Autodesk Fusion 360 part; units mm, degrees
(part 2 of 3)
sketch "스케치1 (3)" plane through (0, 0, 0) normal (0, 0, 1) x (1, 0, 0) in component "rightKey2"
  line L0 (104.5156, 0) -> (228.5, 0)
  line L1 (150.5375, 25.575) -> (136.5375, 25.575)
  line L2 (160.0625, 44.625) -> (146.0625, 44.625)
  line L3 (145.775, 6.525) -> (131.775, 6.525)
  line L4 (145.775, 20.525) -> (145.775, 6.525)
  line L5 (150.825, 6.525) -> (150.825, 20.525)
  line L6 (131.775, 20.525) -> (145.775, 20.525)
  line L7 (126.725, 20.525) -> (126.725, 6.525)
  line L8 (150.5375, 39.575) -> (150.5375, 25.575)
  line L9 (131.4875, 39.575) -> (131.4875, 25.575)
  line L10 (136.5375, 39.575) -> (150.5375, 39.575)
  line L11 (177.0187, 44.625) -> (177.0187, 50.525)
  line L12 (175.5187, 57.225) -> (175.5187, 52.725)
  line L13 (126.725, 82.725) -> (112.725, 82.725)
  line L14 (112.725, 96.725) -> (126.725, 96.725)
  line L15 (164.825, 20.525) -> (164.825, 6.525)
  line L16 (127.0125, 44.625) -> (127.0125, 58.625)
  line L17 (221.975, 58.625) -> (221.975, 44.625)
  line L18 (124.4875, 42.1) -> (124.4875, 61.15)
  line L19 (119.725, 61.15) -> (124.4875, 61.15)
  line L20 (126.725, 6.525) -> (112.725, 6.525)
  line L21 (191.0188, 58.625) -> (191.0188, 52.725)
  line L22 (146.0625, 44.625) -> (146.0625, 58.625)
  line L23 (192.5187, 52.725) -> (192.5187, 57.225)
  line L24 (129.25, 0) -> (129.25, 103.25) construction
  line L25 (177.0187, 52.725) -> (177.0188, 58.625)
  line L26 (207.975, 44.625) -> (207.975, 58.625)
  line L27 (169.875, 6.525) -> (169.875, 20.525)
  line L28 (188.925, 20.525) -> (202.925, 20.525)
  line L29 (175.5188, 46.025) -> (168.7188, 46.025)
  line L30 (162.7313, 25.575) -> (162.7313, 39.575)
  line L31 (141.0125, 58.625) -> (141.0125, 44.625)
  line L32 (160.0625, 58.625) -> (160.0625, 44.625)
  line L33 (207.975, 6.525) -> (207.975, 20.525)
  line L34 (191.0188, 44.625) -> (177.0187, 44.625)
  line L35 (228.5, 103.25) -> (110.2, 103.25)
  line L36 (221.975, 25.575) -> (207.975, 25.575)
  line L37 (176.7313, 39.575) -> (176.7313, 25.575)
  line L38 (202.925, 25.575) -> (188.925, 25.575)
  line L39 (202.925, 6.525) -> (188.925, 6.525)
  line L40 (141.0125, 44.625) -> (127.0125, 44.625)
  line L41 (136.5375, 25.575) -> (136.5375, 39.575)
  line L42 (131.775, 6.525) -> (131.775, 20.525)
  line L43 (112.725, 20.525) -> (126.725, 20.525)
  line L44 (175.5188, 50.525) -> (175.5188, 46.025)
  line L45 (221.975, 39.575) -> (221.975, 25.575)
  line L46 (114.9625, 42.1) -> (124.4875, 42.1)
  line L47 (177.0187, 50.525) -> (175.5188, 50.525)
  line L48 (117.4875, 39.575) -> (131.4875, 39.575)
  line L49 (131.4875, 25.575) -> (117.4875, 25.575)
  line L50 (188.925, 39.575) -> (202.925, 39.575)
  line L51 (162.7313, 39.575) -> (176.7313, 39.575)
  line L52 (177.0188, 58.625) -> (191.0188, 58.625)
  line L53 (177.9, 90.825) -> (179.4, 90.825)
  line L54 (136.25, 63.675) -> (122.25, 63.675)
  line L55 (155.3, 63.675) -> (141.3, 63.675)
  line L56 (207.975, 96.725) -> (221.975, 96.725)
  line L57 (145.775, 82.725) -> (131.775, 82.725)
  line L58 (179.4, 96.725) -> (193.4, 96.725)
  circle A0 centre (225.4, 3.1) radius 1.6
  line L59 (122.25, 63.675) -> (122.25, 77.675)
  line L60 (127.0125, 58.625) -> (141.0125, 58.625)
  line L61 (193.4, 88.625) -> (193.4, 82.725)
  line L62 (136.25, 77.675) -> (136.25, 63.675)
  line L63 (146.0625, 58.625) -> (160.0625, 58.625)
  line L64 (194.9, 84.125) -> (194.9, 88.625)
  line L65 (164.825, 82.725) -> (150.825, 82.725)
  line L66 (207.975, 77.675) -> (221.975, 77.675)
  line L67 (202.925, 39.575) -> (202.925, 25.575)
  line L68 (126.725, 96.725) -> (126.725, 82.725)
  line L69 (179.4, 82.725) -> (179.4, 88.625)
  line L70 (194.9, 95.325) -> (201.7, 95.325)
  line L71 (183.875, 6.525) -> (169.875, 6.525)
  line L72 (199.3187, 46.025) -> (192.5187, 46.025)
  line L73 (160.35, 63.675) -> (160.35, 77.675)
  line L74 (183.875, 20.525) -> (183.875, 6.525)
  line L75 (202.925, 20.525) -> (202.925, 6.525)
  line L76 (145.775, 96.725) -> (145.775, 82.725)
  line L77 (179.4, 90.825) -> (179.4, 96.725)
  circle A1 centre (225.4, 100.15) radius 1.6
  line L78 (194.9, 90.825) -> (194.9, 95.325)
  line L79 (207.975, 39.575) -> (221.975, 39.575)
  line L80 (201.7, 84.125) -> (194.9, 84.125)
  line L81 (122.25, 77.675) -> (136.25, 77.675)
  line L82 (141.3, 77.675) -> (155.3, 77.675)
  line L83 (207.975, 58.625) -> (221.975, 58.625)
  line L84 (164.825, 96.725) -> (164.825, 82.725)
  line L85 (168.7188, 57.225) -> (175.5188, 57.225)
  line L86 (131.775, 82.725) -> (131.775, 96.725)
  line L87 (221.975, 63.675) -> (207.975, 63.675)
  line L88 (131.775, 96.725) -> (145.775, 96.725)
  line L89 (155.3, 77.675) -> (155.3, 63.675)
  line L90 (177.9, 95.325) -> (177.9, 90.825)
  line L91 (150.825, 96.725) -> (164.825, 96.725)
  line L92 (193.4, 96.725) -> (193.4, 90.825)
  line L93 (198.1625, 63.675) -> (184.1625, 63.675)
  line L94 (193.4, 90.825) -> (194.9, 90.825)
  line L95 (174.35, 77.675) -> (174.35, 63.675)
  line L96 (150.825, 82.725) -> (150.825, 96.725)
  line L97 (171.1, 95.325) -> (177.9, 95.325)
  line L98 (221.975, 96.725) -> (221.975, 82.725)
  line L99 (192.5187, 57.225) -> (199.3187, 57.225)
  line L100 (177.9, 84.125) -> (171.1, 84.125)
  line L101 (179.4, 88.625) -> (177.9, 88.625)
  line L102 (141.3, 63.675) -> (141.3, 77.675)
  line L103 (194.9, 88.625) -> (193.4, 88.625)
  line L104 (184.1625, 63.675) -> (184.1625, 77.675)
  line L105 (207.975, 63.675) -> (207.975, 77.675)
  line L106 (198.1625, 77.675) -> (198.1625, 63.675)
  line L107 (221.975, 77.675) -> (221.975, 63.675)
  line L108 (221.975, 82.725) -> (207.975, 82.725)
  line L109 (201.7, 95.325) -> (201.7, 84.125)
  line L110 (193.4, 82.725) -> (179.4, 82.725)
  line L111 (184.1625, 77.675) -> (198.1625, 77.675)
  line L112 (207.975, 82.725) -> (207.975, 96.725)
  line L113 (177.9, 88.625) -> (177.9, 84.125)
  line L114 (171.1, 84.125) -> (171.1, 95.325)
  line L115 (119.725, 80.2) -> (119.725, 61.15)
  line L116 (168.7188, 46.025) -> (168.7188, 57.225)
  line L117 (110.2, 80.2) -> (119.725, 80.2)
  line L118 (169.875, 20.525) -> (183.875, 20.525)
  line L119 (117.4875, 25.575) -> (117.4875, 39.575)
  line L120 (117.4875, 25.575) -> (117.4875, 20.525) construction
  line L121 (191.0188, 50.525) -> (191.0188, 44.625)
  line L122 (228.5, 0) -> (228.5, 103.25)
  line L123 (192.5187, 46.025) -> (192.5187, 50.525)
  line L124 (114.9625, 42.1) -> (114.9625, 23.05)
  line L125 (221.975, 44.625) -> (207.975, 44.625)
  line L126 (207.975, 20.525) -> (221.975, 20.525)
  line L127 (112.725, 82.725) -> (112.725, 96.725)
  line L128 (192.5187, 50.525) -> (191.0188, 50.525)
  line L129 (188.925, 25.575) -> (188.925, 39.575)
  line L130 (112.725, 6.525) -> (112.725, 20.525)
  line L131 (188.925, 6.525) -> (188.925, 20.525)
  line L132 (191.0188, 52.725) -> (192.5187, 52.725)
  line L133 (207.975, 25.575) -> (207.975, 39.575)
  line L134 (199.3187, 57.225) -> (199.3187, 46.025)
  line L135 (110.2, 80.2) -> (110.2, 103.25)
  line L136 (221.975, 6.525) -> (207.975, 6.525)
  line L137 (150.825, 20.525) -> (164.825, 20.525)
  line L138 (114.9625, 23.05) -> (104.5156, 23.05)
  line L139 (160.35, 77.675) -> (174.35, 77.675)
  line L140 (221.975, 20.525) -> (221.975, 6.525)
  line L141 (176.7313, 25.575) -> (162.7313, 25.575)
  line L142 (174.35, 63.675) -> (160.35, 63.675)
  line L143 (164.825, 6.525) -> (150.825, 6.525)
  line L144 (104.5156, 23.05) -> (104.5156, 0)
  line L145 (175.5187, 52.725) -> (177.0187, 52.725)
  circle A2 centre (107.6156, 3.1) radius 1.6
  circle A3 centre (132.35, 3.1) radius 1.6
  circle A4 centre (126.15, 3.1) radius 1.6
  circle A5 centre (126.15, 100.15) radius 1.6
  circle A6 centre (132.35, 100.15) radius 1.6
  circle A7 centre (113.3, 100.15) radius 1.6
  point P0 (225.4, 3.1)
  dimension "d467" = -19.05
  dimension "d468" = 0
  dimension "d471" = -19.05
  dimension "d472" = 0
  dimension "d475" = -19.05
  dimension "d476" = 0
  dimension "d479" = -19.05
  dimension "d480" = 0
  dimension "d483" = -19.05
  dimension "d484" = 0
  dimension "d487" = 0
  dimension "d488" = 19.05
  dimension "d491" = 14
  dimension "d492" = 14
  dimension "d493" = 25.575
  dimension "d494" = 6.525
  dimension "d506" = 14
  dimension "d507" = 14
  dimension "d508" = 19.05
  dimension "d509" = 14
  dimension "d510" = 14
  dimension "d511" = 12.1938
  dimension "d512" = 14
  dimension "d513" = 14
  dimension "d514" = 12.1938
  dimension "d515" = 14
  dimension "d516" = 14
  dimension "d517" = 6.8
  dimension "d518" = 11.2
  dimension "d519" = 1.5
  dimension "d520" = 4.5
  dimension "d521" = 5.9
  dimension "d522" = 19.05
  dimension "d523" = 37.4813
  dimension "d524" = 14
  dimension "d525" = 14
  dimension "d526" = 16.9563
  dimension "d527" = 14
  dimension "d528" = 14
  dimension "d529" = 19.05
  dimension "d530" = 30.3375
  dimension "d531" = 14
  dimension "d532" = 14
  dimension "d533" = 9.8125
  dimension "d534" = 14
  dimension "d535" = 14
  dimension "d536" = 6.8
  dimension "d537" = 11.2
  dimension "d538" = 1.5
  dimension "d539" = 4.5
  dimension "d540" = 5.9
  dimension "d541" = 19.05
  dimension "d542" = 35.1
  dimension "d543" = 14
  dimension "d544" = 14
  dimension "d545" = 14.575
  dimension "d546" = 3.2
  dimension "d547" = 3.1
  dimension "d548" = 3.1
  dimension "d549" = 3.2
  dimension "d550" = 3.1
  dimension "d555" = 14
  dimension "d556" = 14
  dimension "d557" = 6.525
  dimension "d558" = 10.4469
  dimension "d559" = 23.05
  dimension "d561" = 19.05
  dimension "d562" = 19.05
  dimension "d563" = 9.525
  dimension "d564" = 4.7625
  dimension "d565" = 9.525
  dimension "d566" = 23.05
  dimension "d622" = 228.5
  dimension "d623" = 123.9844
  dimension "d624" = 103.25
  dimension "d625" = 3.2
  dimension "d626" = 3.1
  dimension "d627" = 3.2
  dimension "d628" = 3.2
  dimension "d629" = 3.1
  dimension "d630" = 3.1
  dimension "d631" = 3.2
  dimension "d632" = 3.2
  dimension "d633" = 3.2
  dimension "d634" = 3.1
  dimension "d635" = 3.1
  dimension "d637" = 3.1
  dimension "d638" = 99.25
  constraint horizontal L0
  constraint vertical L122
  constraint horizontal L35
  constraint horizontal L28
  constraint vertical L75
  constraint horizontal L39
  constraint vertical L131
  constraint horizontal L50
  constraint vertical L67
  constraint horizontal L38
  constraint vertical L129
  constraint vertical L39.start L38.start
  constraint horizontal L51
  constraint vertical L37
  constraint horizontal L141
  constraint vertical L30
  constraint horizontal L37.end L38.end
  constraint horizontal L10
  constraint vertical L8
  constraint horizontal L1
  constraint vertical L41
  constraint horizontal L1.start L30.start
  constraint horizontal L52
  constraint vertical L21
  constraint horizontal L34
  constraint vertical L11
  constraint horizontal L85
  constraint vertical L12
  constraint horizontal L29
  constraint vertical L116
  constraint horizontal L145
  constraint horizontal L128
  constraint horizontal L99
  constraint vertical L134
  constraint horizontal L72
  constraint vertical L123
  constraint collinear L12 L44
  constraint coincident L11.end L128
  constraint collinear L11 L25
  constraint coincident L21.end L145
  constraint collinear L21 L121
  constraint collinear L23 L123
  constraint equal L85 L99
  constraint equal L116 L134
  constraint equal L12 L23
  constraint equal L12 L44
  constraint horizontal L63
  constraint vertical L32
  constraint horizontal L2
  constraint vertical L22
  constraint horizontal L2.start L11.start
  constraint horizontal L111
  constraint vertical L106
  constraint horizontal L93
  constraint vertical L104
  constraint horizontal L139
  constraint vertical L95
  constraint horizontal L142
  constraint vertical L73
  constraint horizontal L93.end L95.end
  constraint horizontal L58
  constraint vertical L92
  constraint horizontal L110
  constraint vertical L69
  constraint horizontal L97
  constraint vertical L90
  constraint horizontal L100
  constraint vertical L114
  constraint horizontal L53
  constraint horizontal L103
  constraint horizontal L70
  constraint vertical L109
  constraint horizontal L80
  constraint vertical L64
  constraint collinear L90 L113
  constraint coincident L69.end L103
  constraint collinear L69 L77
  constraint coincident L92.end L53
  constraint collinear L61 L92
  constraint collinear L64 L78
  constraint collinear L101 L103
  constraint collinear L53 L94
  constraint equal L70 L97
  constraint equal L109 L114
  constraint equal L78 L90
  constraint equal L90 L113
  constraint horizontal L91
  constraint vertical L84
  constraint horizontal L65
  constraint vertical L96
  constraint horizontal L69.start L65.start
  constraint vertical A1.centre P0
  constraint horizontal L126
  constraint vertical L140
  constraint horizontal L136
  constraint vertical L33
  constraint horizontal L39.start L33.start
  constraint coincident L120.end L43
  constraint perpendicular L43 L120
  constraint perpendicular L124 L138
  constraint perpendicular L18 L54
  constraint perpendicular L18 L19
  constraint perpendicular L19 L115
  constraint perpendicular L35 L135
  constraint perpendicular L0 L144
  constraint perpendicular L46 L124
  constraint perpendicular L18 L46
  constraint perpendicular L115 L117
  constraint coincident L24.end L35
  constraint coincident L24.start L0
  constraint equal L132 L145
  constraint equal L47 L128
  constraint equal L53 L94
  constraint horizontal P0 A2.centre
  constraint horizontal P0 A3.centre
  constraint horizontal A3.centre A4.centre
  constraint horizontal A5.centre A6.centre
  constraint horizontal A1.centre A6.centre
  constraint horizontal origin L0.end
  constraint vertical L24
  constraint horizontal A1.centre A7.centre
  measures "d491" distance of L28.start L28.end
  measures "d492" distance of L39.end L28.start
  measures "d493" horizontal distance of L0.end L39.start
  measures "d494" vertical distance of L0.end L39.start
  measures "d506" distance of L50.start L50.end
  measures "d507" distance of L50.start L38.end
  measures "d508" distance of L39.start L38.start
  measures "d509" distance of L30.end L37.start
  measures "d510" distance of L30.start L30.end
  measures "d511" distance of L37.end L38.end
  measures "d512" distance of L10.start L8.start
  measures "d513" distance of L10.start L1.end
  measures "d514" distance of L1.start L30.start
  measures "d515" distance of L21.start L25.end
  measures "d516" distance of L11.start L25.end
  measures "d517" distance of L85.start L12.start
  measures "d518" distance of L29.end L85.start
  measures "d519" distance of L25.start L12.end
  measures "d520" distance of L12.end L12.start
  measures "d521" distance of L25.start L25.end
  measures "d522" vertical distance of L34.start L38.start
  measures "d523" distance of L34.start L122
  measures "d524" distance of L32.start L22.end
  measures "d525" distance of L22.end L2.end
  measures "d526" distance of L2.start L11.start
  measures "d527" distance of L104.end L106.start
  measures "d528" distance of L93.end L104.end
  measures "d529" vertical distance of L93.start L34.start
  measures "d530" distance of L93.start L122
  measures "d531" distance of L73.end L95.start
  measures "d532" distance of L73.end L73.start
  measures "d533" distance of L93.end L95.end
  measures "d534" distance of L58.end L58.start
  measures "d535" distance of L69.start L58.start
  measures "d536" distance of L90.start L97.start
  measures "d537" distance of L100.end L97.start
  measures "d538" distance of L53.end L53.start
  measures "d539" distance of L90.start L53.start
  measures "d540" distance of L53.end L58.start
  measures "d541" vertical distance of L93.start L61.end
  measures "d542" distance of L61.end L122
  measures "d543" distance of L84.start L91.start
  measures "d544" distance of L91.start L65.end
  measures "d545" horizontal distance of L69.start L65.start
  measures "d546" diameter of A0
  measures "d547" vertical distance of P0 L0.end
  measures "d548" horizontal distance of P0 L0.end
  measures "d549" diameter of A1
  measures "d550" vertical distance of A1.centre L35.start
  measures "d555" distance of L33.end L126.end
  measures "d556" distance of L33.end L33.start
  measures "d557" horizontal distance of L0.end L136.start
  measures "d558" distance of L124.end L138.end
  measures "d559" distance of L0.start L138.end
  measures "d561" distance of L124.end L46.start
  measures "d562" distance of L18.start L18.end
  measures "d563" distance of L46.start L18.start
  measures "d564" distance of L19.start L18.end
  measures "d565" distance of L117.start L115.start
  measures "d566" distance of L35.end L117.start
  measures "d622" distance of L0.end origin
  measures "d623" distance of L0.end L0.start
  measures "d624" distance of L35.start L0.end
  measures "d625" diameter of A2
  measures "d626" horizontal distance of L0.start A2.centre
  measures "d627" diameter of A3
  measures "d628" diameter of A4
  measures "d629" horizontal distance of L24.start A4.centre
  measures "d630" horizontal distance of L24.start A3.centre
  measures "d631" diameter of A6
  measures "d632" diameter of A5
  measures "d633" diameter of A7
  measures "d634" horizontal distance of L24.end A6.centre
  measures "d635" horizontal distance of L24.end A5.centre
  measures "d637" horizontal distance of L35.end A7.centre
  measures "d638" distance of L24.start L0.end
extrude "돌출1''" add sketch "스케치1 (3)" along normal blind 3 separate body makes body 3 in component "rightKey2"
sketch "스케치2 (3)" plane through (0, 0, 3) normal (0, 0, 1) x (-1, 0, 0) in component "rightKey2"
  circle A0 centre (-113.3, -100.15) radius 1.6
  circle A1 centre (-126.15, -100.15) radius 1.6
  circle A2 centre (-132.35, -100.15) radius 1.6
  circle A3 centre (-225.4, -100.15) radius 1.6
  circle A4 centre (-225.4, -3.1) radius 1.6
  circle A5 centre (-132.35, -3.1) radius 1.6
  circle A6 centre (-126.15, -3.1) radius 1.6
  circle A7 centre (-107.6156, -3.1) radius 1.6
  circle A8 centre (-107.6156, -3.1) radius 3
  circle A9 centre (-126.15, -3.1) radius 3
  circle A10 centre (-132.35, -3.1) radius 3
  circle A11 centre (-225.4, -3.1) radius 3
  circle A12 centre (-225.4, -100.15) radius 3
  circle A13 centre (-132.35, -100.15) radius 3
  circle A14 centre (-126.15, -100.15) radius 3
  circle A15 centre (-113.3, -100.15) radius 3
  dimension "d641" = 6
  dimension "d642" = 6
  dimension "d643" = 6
  dimension "d644" = 6
  dimension "d645" = 6
  dimension "d646" = 6
  dimension "d647" = 6
  dimension "d649" = 6
  constraint concentric A7 A8
  constraint concentric A6 A9
  constraint concentric A5 A10
  constraint concentric A4 A11
  constraint concentric A3 A12
  constraint concentric A2 A13
  constraint concentric A1 A14
  constraint concentric A0 A15
  measures "d641" diameter of A8
  measures "d642" diameter of A9
  measures "d643" diameter of A10
  measures "d644" diameter of A11
  measures "d645" diameter of A12
  measures "d646" diameter of A13
  measures "d647" diameter of A14
  measures "d649" diameter of A15
extrude "돌출2''" cut sketch "스케치2 (3)" against normal blind 1.75 bodies 3 in component "rightKey2"
fillet "모깎기1'" radius 3.1 2 edges at (228.5, 0, 1.5) (228.5, 103.25, 1.5) on bodies 3 in component "rightKey2"
extrude "돌출3'" add sketch "스케치1 (2)" along normal blind 3 separate body contours L2 L10 L11 L43 L44 L45 L46 L47 L48 L49 L50 L51 makes body 4 in component "rightKey1"
sketch "스케치3 (3)" plane through (0, 0, 3) normal (0, 0, 1) x (-1, 0, 0) in component "rightKey1"
  circle A0 centre (-107.1, -100.15) radius 1.6
  circle A1 centre (-101.4156, -3.1) radius 1.6
  circle A2 centre (-33.1, -3.1) radius 1.6
  circle A3 centre (-33.1, -100.15) radius 1.6
  circle A4 centre (-107.1, -100.15) radius 3
  circle A5 centre (-33.1, -100.15) radius 3
  circle A6 centre (-33.1, -3.1) radius 3
  circle A7 centre (-101.4156, -3.1) radius 3
  point P0 (-33.1, -100.15)
  dimension "d656" = 6
  dimension "d657" = 6
  dimension "d658" = 6
  dimension "d659" = 6
  constraint concentric A0 A4
  constraint concentric A3 A5
  constraint concentric A2 A6
  constraint concentric A1 A7
  measures "d656" diameter of A4
  measures "d657" diameter of A5
  measures "d658" diameter of A6
  measures "d659" diameter of A7
extrude "돌출4'" cut sketch "스케치3 (3)" against normal blind 1.75 bodies 4 in component "rightKey1"
fillet "모깎기2" radius 3.1 2 edges at (30, 0, 1.5) (30, 103.25, 1.5) on bodies 4 in component "rightKey1"
sketch "스케치1 (4)" plane through (0, 0, 0) normal (0, 0, 1) x (1, 0, 0) in component "rightBody1"
  line L0 (30, 103.25) -> (30, 0)
  line L1 (228.5, 3.1) -> (228.5, 100.15)
  circle A0 centre (126.15, 3.1) radius 1.6
  circle A1 centre (132.35, 3.1) radius 1.6
  circle A2 centre (126.15, 100.15) radius 1.6
  circle A3 centre (132.35, 100.15) radius 1.6
  line L2 (126.15, 3.1) -> (132.35, 3.1) construction
  line L3 (126.15, 100.15) -> (132.35, 100.15) construction
  line L4 (129.25, 100.15) -> (129.25, 3.1)
  line L5 (30, 0) -> (129.25, 0)
  line L6 (129.25, 0) -> (129.25, 3.1)
  line L7 (30, 103.25) -> (129.25, 103.25)
  line L8 (129.25, 103.25) -> (129.25, 100.15)
  line L9 (30, 0) -> (30, 103.25)
  line L10 (30, 103.25) -> (30, 0)
  circle A4 centre (113.3, 100.15) radius 1.6
  circle A5 centre (107.1, 100.15) radius 1.6
  circle A6 centre (33.1, 100.15) radius 1.6
  circle A7 centre (33.1, 3.1) radius 1.6
  circle A8 centre (101.4156, 3.1) radius 1.6
  circle A9 centre (107.6156, 3.1) radius 1.6
  circle A10 centre (126.15, 3.1) radius 1.6
  circle A11 centre (126.15, 100.15) radius 1.6
  circle A12 centre (33.1, 100.15) radius 1.5
  circle A13 centre (107.1, 100.15) radius 1.5
  circle A14 centre (113.3, 100.15) radius 1.5
  circle A15 centre (126.15, 100.15) radius 1.5
  circle A16 centre (126.15, 3.1) radius 1.5
  circle A17 centre (107.6156, 3.1) radius 1.5
  circle A18 centre (101.4156, 3.1) radius 1.5
  circle A19 centre (33.1, 3.1) radius 1.5
  line L11 (129.25, 2.5) -> (128.448, 2.5)
  arc A20 (128.448, 2.5) -> (123.852, 2.5) centre (126.15, 3.1) ccw
  line L12 (123.852, 2.5) -> (109.9136, 2.5)
  arc A21 (109.9136, 2.5) -> (105.3177, 2.5) centre (107.6156, 3.1) ccw
  line L13 (105.3177, 2.5) -> (103.7136, 2.5)
  arc A22 (103.7136, 2.5) -> (99.1177, 2.5) centre (101.4156, 3.1) ccw
  arc A23 (35.398, 2.5) -> (32.5, 5.398) centre (33.1, 3.1) ccw
  line L14 (99.1177, 2.5) -> (35.398, 2.5)
  line L15 (32.5, 5.398) -> (32.5, 97.852)
  arc A24 (32.5, 97.852) -> (35.398, 100.75) centre (33.1, 100.15) ccw
  arc A25 (104.802, 100.75) -> (109.398, 100.75) centre (107.1, 100.15) ccw
  line L16 (35.398, 100.75) -> (104.802, 100.75)
  line L17 (109.398, 100.75) -> (111.002, 100.75)
  arc A26 (111.002, 100.75) -> (115.598, 100.75) centre (113.3, 100.15) ccw
  arc A27 (123.852, 100.75) -> (128.448, 100.75) centre (126.15, 100.15) ccw
  line L18 (115.598, 100.75) -> (123.852, 100.75)
  line L19 (128.448, 100.75) -> (129.25, 100.75)
  line L20 (30, 0) -> (104.5156, 0) construction
  dimension "d664" = 3
  dimension "d665" = 3
  dimension "d666" = 3
  dimension "d667" = 3
  dimension "d668" = 3
  dimension "d669" = 3
  dimension "d670" = 3
  dimension "d671" = 3
  dimension "d672" = 4.75
  dimension "d674" = 4.75
  dimension "d675" = 4.75
  dimension "d676" = 4.75
  dimension "d677" = 4.75
  dimension "d678" = 4.75
  dimension "d679" = 4.75
  dimension "d680" = 2.5
  dimension "d682" = 2.5
  dimension "d683" = 2.5
  dimension "d686" = 4.75
  dimension "d687" = 2.5
  dimension "d688" = 2.5
  dimension "d689" = 2.5
  dimension "d690" = 2.5
  constraint coincident A0.centre L2.start
  constraint coincident A1.centre L2.end
  constraint coincident A2.centre L3.start
  constraint coincident A3.centre L3.end
  constraint midpoint L3 L4.start
  constraint midpoint L2 L4.end
  constraint coincident L0.end L5.start
  constraint perpendicular L4 L5
  constraint perpendicular L2 L6
  constraint coincident L0.start L7.start
  constraint perpendicular L0 L7
  constraint perpendicular L3 L8
  constraint concentric A6 A12
  constraint concentric A5 A13
  constraint concentric A4 A14
  constraint concentric A11 A15
  constraint concentric A10 A16
  constraint concentric A9 A17
  constraint concentric A8 A18
  constraint concentric A7 A19
  constraint concentric A19 A23
  constraint concentric A13 A25
  constraint concentric A4 A26
  constraint concentric A11 A27
  constraint concentric A16 A20
  constraint concentric A9 A21
  constraint concentric A18 A22
  constraint coincident L6 L11.start
  constraint perpendicular L10 L11
  constraint coincident L8 L19.end
  constraint concentric A12 A24
  constraint horizontal L16
  constraint coincident A25.end L16
  constraint horizontal L17
  constraint horizontal L18
  constraint coincident A27.end L18
  constraint horizontal L19
  constraint horizontal L12
  constraint horizontal L13
  constraint horizontal L14
  constraint vertical L15
  measures "d664" diameter of A12
  measures "d665" diameter of A13
  measures "d666" diameter of A14
  measures "d667" diameter of A15
  measures "d668" diameter of A16
  measures "d669" diameter of A17
  measures "d670" diameter of A18
  measures "d671" diameter of A19
  measures "d672" diameter of A23
  measures "d674" diameter of A25
  measures "d675" diameter of A26
  measures "d676" diameter of A27
  measures "d677" diameter of A20
  measures "d678" diameter of A21
  measures "d679" diameter of A22
  measures "d680" distance of L5.end L11.start
  measures "d682" distance of L9 A23.end
  measures "d683" distance of L7 A24.end
  measures "d686" diameter of A24
  measures "d687" distance of L7 A26.end
  measures "d688" distance of L5 L12.end
  measures "d689" distance of L5 A21.end
  measures "d690" distance of A22.end L20
move_face "면 간격띄우기1" offset 0.2 9 faces at (111.4802, 23.05, 2) (118.1375, 42.1, 1) (121.3125, 61.15, 1) (113.375, 80.2, 1) (104.5156, 15.3667, 1) (114.9625, 35.75, 1) (124.4875, 48.45, 1) (119.725, 73.85, 1) (110.2, 87.8833, 1) on bodies 3 in component "rightKey2"
extrude "돌출1'''" add sketch "스케치1 (4)" against normal blind 15 separate body contours L0 L5 L6 L7 L8 L9 L10 L11 A20 L12 A21 L13 A22 A23 L14 L15 A24 A25 L16 L17 A26 A27 L18 L19 | L4 L6 L8 L11 A20 L12 A21 L13 A22 A23 L14 L15 A24 A25 L16 L17 A26 A27 L18 L19 | A0 A10 | A2 A11 | A4 | A5 | A6 | A7 | A8 | A9 | A12 | A13 | A14 | A15 | A16 | A17 | A18 | A19 makes body 5 in component "rightBody1"
extrude "돌출2'''" cut sketch "스케치1 (4)" against normal blind 13 contours L4 L6 L8 L11 A20 L12 A21 L13 A22 A23 L14 L15 A24 A25 L16 L17 A26 A27 L18 L19 bodies 5 in component "rightBody1"
extrude "돌출3''" cut sketch "스케치1 (4)" against normal blind 10 contours A12 | A13 | A14 | A15 | A16 | A17 | A18 | A19 bodies 5 in component "rightBody1"
sketch "스케치1 (5)" plane through (0, 0, 0) normal (0, 0, 1) x (1, 0, 0) in component "rightBody2"
  line L0 (104.3156, 0) -> (225.4, 0)
  line L1 (228.5, 3.1) -> (228.5, 100.15)
  line L2 (129.25, 100.15) -> (129.25, 3.1)
  line L3 (129.25, 0) -> (129.25, 3.1)
  circle A0 centre (132.35, 100.15) radius 1.6
  circle A1 centre (225.4, 100.15) radius 1.6
  circle A2 centre (225.4, 3.1) radius 1.6
  circle A3 centre (132.35, 3.1) radius 1.6
  line L4 (129.25, 0) -> (228.5, 0)
  line L5 (228.5, 0) -> (228.5, 103.25)
  line L6 (228.5, 103.25) -> (129.25, 103.25)
  line L7 (129.25, 103.25) -> (129.25, 0)
  circle A4 centre (132.35, 100.15) radius 1.5
  circle A5 centre (225.4, 100.15) radius 1.5
  circle A6 centre (132.35, 3.1) radius 1.5
  circle A7 centre (225.4, 3.1) radius 1.5
  arc A8 (130.052, 100.75) -> (134.648, 100.75) centre (132.35, 100.15) ccw
  line L8 (129.25, 100.75) -> (130.052, 100.75)
  arc A9 (134.648, 2.5) -> (130.052, 2.5) centre (132.35, 3.1) ccw
  line L9 (129.25, 2.5) -> (130.052, 2.5)
  arc A10 (226, 5.398) -> (223.102, 2.5) centre (225.4, 3.1) ccw
  line L10 (134.648, 2.5) -> (223.102, 2.5)
  line L11 (226, 4.5832) -> (226, 4.4748)
  arc A11 (223.102, 100.75) -> (226, 97.852) centre (225.4, 100.15) ccw
  line L12 (134.648, 100.75) -> (223.102, 100.75)
  line L13 (226, 97.852) -> (226, 5.398)
  point P0 (129.25, 103.25)
  dimension "d697" = 103.25
  dimension "d698" = 99.25
  dimension "d699" = 3
  dimension "d700" = 3
  dimension "d701" = 3
  dimension "d702" = 3
  dimension "d703" = 4.75
  dimension "d704" = 4.75
  dimension "d705" = 4.75
  dimension "d706" = 4.75
  dimension "d707" = 2.5
  dimension "d708" = 2.5
  dimension "d710" = 2.5
  dimension "d711" = 2.5
  constraint horizontal L4
  constraint vertical L5
  constraint horizontal L6
  constraint vertical L7
  constraint coincident L3.start L4.start
  constraint concentric A0 A4
  constraint concentric A1 A5
  constraint concentric A3 A6
  constraint concentric A2 A7
  constraint concentric A2 A10
  constraint concentric A3 A9
  constraint concentric A0 A8
  constraint concentric A5 A11
  constraint coincident L7 L8.start
  constraint perpendicular L5 L8
  constraint coincident A8.end L8
  constraint collinear L8 L12
  constraint coincident L3 L9.start
  constraint perpendicular L5 L9
  constraint coincident A9.start L9
  constraint collinear L9 L10
  constraint coincident A7 L11.end
  constraint coincident A2 L11.start
  measures "d697" distance of L4.end L5.end
  measures "d698" distance of L3.start L4.end
  measures "d699" diameter of A4
  measures "d700" diameter of A5
  measures "d701" diameter of A6
  measures "d702" diameter of A7
  measures "d703" diameter of A10
  measures "d704" diameter of A9
  measures "d705" diameter of A8
  measures "d706" diameter of A11
  measures "d707" distance of P0 L8.start
  measures "d708" distance of L3.start L9.start
  measures "d710" distance of L5 A10.start
  measures "d711" distance of L5 A11.end
extrude "돌출1''''" add sketch "스케치1 (5)" against normal blind 15 separate body contours L0 L1 L3 L4 L5 L6 L7 A8 L8 A9 L9 A10 L10 A11 L12 L13 | L2 L3 L7 A8 L8 A9 L9 A10 L10 A11 L12 L13 | A0 | A1 | A2 | A3 | A4 | A5 | A6 | A7 makes body 6 in component "rightBody2"
extrude "돌출2''''" cut sketch "스케치1 (5)" against normal blind 13 contours L2 L3 L7 A8 L8 A9 L9 A10 L10 A11 L12 L13 bodies 6 in component "rightBody2"
extrude "돌출3'''" cut sketch "스케치1 (5)" against normal blind 10 contours A4 | A5 | A6 | A7 bodies 6 in component "rightBody2"
sketch "스케치2 (4)" plane through (0, 0, -13) normal (0, 0, 1) x (-1, 0, 0) in component "rightBody1"
  line L0 (-35.398, -100.75) -> (-104.802, -100.75)
  line L1 (-40.398, -85.75) -> (-52.398, -85.75)
  line L2 (-52.398, -85.75) -> (-52.398, -84.75)
  line L3 (-52.398, -84.75) -> (-40.398, -84.75)
  line L4 (-40.398, -84.75) -> (-40.398, -85.75)
  line L5 (-65.398, -65.15) -> (-83.398, -65.15)
  line L6 (-83.398, -65.15) -> (-83.398, -64.15)
  line L7 (-83.398, -64.15) -> (-65.398, -64.15)
  line L8 (-65.398, -64.15) -> (-65.398, -65.15)
  point P0 (-35.398, -100.75)
  dimension "d718" = 12
  dimension "d719" = 1
  dimension "d720" = 5
  dimension "d721" = 15
  dimension "d722" = 18
  dimension "d723" = 1
  dimension "d724" = 30
  dimension "d725" = 35.6
  constraint horizontal L1
  constraint vertical L2
  constraint horizontal L3
  constraint vertical L4
  constraint horizontal L5
  constraint vertical L6
  constraint horizontal L7
  constraint vertical L8
  measures "d718" distance of L1.start L1.end
  measures "d719" distance of L1.start L3.end
  measures "d720" horizontal distance of L1.start P0
  measures "d721" vertical distance of L1.start P0
  measures "d722" distance of L5.start L5.end
  measures "d723" distance of L5.start L7.end
  measures "d724" horizontal distance of P0 L7.end
  measures "d725" vertical distance of P0 L5.start
extrude "돌출4''" add sketch "스케치2 (4)" along normal blind 2 bodies 5 in component "rightBody1"
sketch "스케치3 (4)" plane through (83.398, 0, 0) normal (1, 0, 0) x (0, 1, 0) in component "rightBody1"
  line L0 (65.15, -11) -> (64.15, -11)
  line L1 (64.15, -11) -> (64.15, -10.4348)
  line L2 (64.8262, -10.1455) -> (65.7214, -11)
  line L3 (65.7214, -11) -> (64.15, -11)
  arc A0 (64.8262, -10.1455) -> (64.15, -10.4348) centre (64.55, -10.4348) ccw
  point P0 (65.7214, -11)
  point P1 (64.15, -11)
  point P2 (64.15, -9.5)
  dimension "d728" = 0.4
  constraint coincident P1 L0.end
  constraint coincident P0 L2.end
  constraint tangent L1 A0
  constraint tangent L2 A0
  measures "d728" radius of A0
extrude "돌출5'" add sketch "스케치3 (4)" against normal blind 18 bodies 5 in component "rightBody1"
extrude "돌출1'''''" add sketch "스케치1 (2)" along normal blind 3 separate body contours L2 L10 L11 L43 L44 L45 L46 L47 L48 L49 L50 L51 makes body 7 in component "rightKey1"
sketch "스케치2 (5)" plane through (0, 0, 3) normal (0, 0, 1) x (-1, 0, 0) in component "rightKey1"
  circle A0 centre (-33.1, -100.15) radius 1.6
  circle A1 centre (-107.1, -100.15) radius 1.6
  circle A2 centre (-33.1, -3.1) radius 1.6
  circle A3 centre (-101.4156, -3.1) radius 1.6
  circle A4 centre (-33.1, -100.15) radius 3
  circle A5 centre (-107.1, -100.15) radius 3
  circle A6 centre (-33.1, -3.1) radius 3
  circle A7 centre (-101.4156, -3.1) radius 3
  dimension "d614" = 6
  dimension "d615" = 6
  dimension "d616" = 6
  dimension "d617" = 6
  constraint concentric A0 A4
  constraint concentric A1 A5
  constraint concentric A2 A6
  constraint concentric A3 A7
  measures "d614" diameter of A4
  measures "d615" diameter of A5
  measures "d616" diameter of A6
  measures "d617" diameter of A7
extrude "돌출2'''''" cut sketch "스케치2 (5)" against normal blind 1.75 bodies 7 in component "rightKey1"
fillet "모깎기1''" radius 3.1 2 edges at (30, 0, 1.5) (30, 103.25, 1.5) on bodies 7 in component "rightKey1"
sketch "스케치4 (2)" plane through (0, 103.25, 0) normal (0, 1, 0) x (-1, 0, 0) in component "rightBody1"
  line L0 (-65.398, -13) -> (-83.398, -13)
  line L1 (-40.398, -13) -> (-52.398, -13)
  circle A0 centre (-48.398, -10) radius 3.2
  line L2 (-71.498, -7.9) -> (-77.298, -7.9)
  arc A1 (-77.298, -7.9) -> (-77.298, -11.5) centre (-77.298, -9.7) ccw
  line L3 (-77.298, -11.5) -> (-71.498, -11.5)
  arc A2 (-71.498, -11.5) -> (-71.498, -7.9) centre (-71.498, -9.7) ccw
  line L4 (-71.498, -9.7) -> (-77.298, -9.7) construction
  line L5 (-83.398, -13) -> (-65.398, -13)
  line L6 (-71.498, -6.1) -> (-77.298, -6.1)
  arc A3 (-77.298, -6.1) -> (-77.298, -13.3) centre (-77.298, -9.7) ccw
  line L7 (-77.298, -13.3) -> (-71.498, -13.3)
  arc A4 (-71.498, -13.3) -> (-71.498, -6.1) centre (-71.498, -9.7) ccw
  line L8 (-71.498, -9.7) -> (-77.298, -9.7) construction
  line L9 (-62.398, -6.8) -> (-56.198, -6.8)
  line L10 (-56.198, -6.8) -> (-56.198, -13)
  line L11 (-56.198, -13) -> (-62.398, -13)
  line L12 (-62.398, -13) -> (-62.398, -6.8)
  line L13 (-62.398, -6.8) -> (-61.898, -6.8)
  line L14 (-61.898, -6.8) -> (-61.898, -13)
  line L15 (-61.898, -13) -> (-62.398, -13)
  line L16 (-62.398, -13) -> (-62.398, -6.8)
  line L17 (-56.198, -6.8) -> (-56.698, -6.8)
  line L18 (-56.698, -6.8) -> (-56.698, -13)
  line L19 (-56.698, -13) -> (-56.198, -13)
  line L20 (-56.198, -13) -> (-56.198, -6.8)
  point P0 (-35.398, -13)
  point P1 (-65.398, -13)
  dimension "d731" = 6.4
  dimension "d732" = 3
  dimension "d733" = 13
  dimension "d734" = 5.8
  dimension "d735" = 1.8
  dimension "d736" = 3.3
  dimension "d737" = 6.1
  dimension "d738" = 3.6
  dimension "d928" = 6.2
  dimension "d929" = 6.2
  dimension "d930" = 3
  dimension "d932" = 0.5
  dimension "d933" = 0.5
  constraint tangent L2 A1
  constraint tangent A1 L3
  constraint parallel L2 L3
  constraint tangent L3 A2
  constraint tangent L2 A2
  constraint horizontal L4
  constraint tangent L6 A3
  constraint tangent A3 L7
  constraint parallel L6 L7
  constraint tangent L7 A4
  constraint tangent L6 A4
  constraint coincident A1.centre L4.end
  constraint parallel L4 L8
  constraint coincident A2.centre L4.start
  constraint horizontal L9
  constraint vertical L10
  constraint horizontal L11
  constraint vertical L12
  constraint collinear L0 L11
  constraint horizontal L13
  constraint vertical L14
  constraint horizontal L15
  constraint vertical L16
  constraint horizontal L17
  constraint vertical L18
  constraint horizontal L19
  constraint vertical L20
  measures "d731" diameter of A0
  measures "d732" distance of L1 A0.centre
  measures "d733" horizontal distance of A0.centre P0
  measures "d734" distance of A2.centre A1.centre
  measures "d735" radius of A1
  measures "d736" distance of A1.centre L5
  measures "d737" horizontal distance of A2.centre P1
  measures "d738" radius of A3
  measures "d928" distance of L9.start L9.end
  measures "d929" distance of L9.start L11.end
  measures "d930" horizontal distance of L0.start L11.end
  measures "d932" distance of L9.start L13.end
  measures "d933" distance of L9.end L17.end
extrude "돌출6'" cut sketch "스케치4 (2)" against normal blind 2.5 contours L1 A0 | L2 A1 L3 A2 | L9 L11 L12 L13 L14 L15 L16 | L9 L10 L11 L17 L18 L19 L20 picked at (-49.417, -9.8038) bodies 5 in component "rightBody1"
extrude "돌출7'" cut sketch "스케치4 (2)" against normal blind 1.5 contours L0 L5 L6 A3 A4 | L9 L11 L14 L18 bodies 5 in component "rightBody1"
sketch "스케치1 (6)" plane through (0, 0, 0) normal (0, 0, 1) x (1, 0, 0) in component "tempJoin"
  line L0 (0, -28.5627) -> (6.2, -28.5627)
  arc A0 (6.2, -28.5627) -> (6.2, -23.8127) centre (6.2, -26.1877) ccw
  line L1 (6.2, -23.8127) -> (0, -23.8127)
  arc A1 (0, -23.8127) -> (0, -28.5627) centre (0, -26.1877) ccw
  line L2 (0, -26.1877) -> (6.2, -26.1877) construction
  circle A2 centre (0, -26.1877) radius 1.5
  circle A3 centre (6.2, -26.1877) radius 1.5
  dimension "d743" = 4.75
  dimension "d744" = 3
  dimension "d745" = 3
  constraint tangent L0 A0
  constraint tangent A0 L1
  constraint parallel L0 L1
  constraint tangent L1 A1
  constraint tangent L0 A1
  constraint horizontal L2
  constraint concentric A1 A2
  constraint concentric A0 A3
  measures "d743" diameter of A0
  measures "d744" diameter of A2
  measures "d745" diameter of A3
extrude "돌출1''''''" add sketch "스케치1 (6)" along normal blind 5 separate body makes body 8 in component "tempJoin"
fillet "모깎기1'''" radius 3.1 2 edges at (228.5, 0, -7.5) (228.5, 103.25, -7.5) on bodies 6 in component "rightBody2"
fillet "모깎기1''''" radius 3.1 2 edges at (30, 103.25, -7.5) (30, 0, -7.5) on bodies 5 in component "rightBody1"
sketch "스케치5" plane through (0, 0, -13) normal (0, 0, 1) x (-1, 0, 0) in component "rightBody1"
  line L0 (-124.4875, -42.1) -> (-124.4875, -61.15)
  line L1 (-129.25, -103.25) -> (-129.25, 0)
  circle A0 centre (-124.4875, -51.625) radius 2.1
  line L2 (-83.8625, -58.625) -> (-83.8625, -44.625)
  line L3 (-88.9125, -44.625) -> (-88.9125, -58.625)
  line L4 (-83.8625, -51.625) -> (-88.9125, -51.625) construction
  circle A1 centre (-86.3875, -51.625) radius 2.1
  dimension "d752" = 4.2
  dimension "d765" = 4.2
  constraint midpoint L0 A0.centre
  constraint midpoint L2 L4.start
  constraint midpoint L3 L4.end
  constraint midpoint L4 A1.centre
  measures "d752" diameter of A0
  measures "d765" diameter of A1
extrude "돌출8" add sketch "스케치5" along normal blind 13 bodies 5 in component "rightBody1"
move_face "면 간격띄우기1'" offset 0.2 1 faces at (129.25, 0.8333, -9.3333) on bodies 6 in component "rightBody2"
sketch "스케치3 (5)" plane through (0, 0, -13) normal (0, 0, 1) x (-1, 0, 0) in component "rightBody2"
  line L0 (-160.0625, -58.625) -> (-160.0625, -44.625)
  line L1 (-168.7188, -46.025) -> (-168.7188, -57.225)
  line L2 (-160.0625, -51.625) -> (-168.7188, -51.625) construction
  circle A0 centre (-164.3906, -51.625) radius 2.5
  dimension "d766" = 5
  constraint midpoint L0 L2.start
  constraint midpoint L1 L2.end
  constraint midpoint L2 A0.centre
  measures "d766" diameter of A0
extrude "돌출4'''" add sketch "스케치3 (5)" along normal blind 13 bodies 6 in component "rightBody2"
extrude "돌출8'" add sketch "스케치2 (2)" along normal blind 13 contours A0 | A1 | A2 | A3 | A4 bodies 2 in component "leftBody1"
sketch "스케치1 (7)" plane through (228.5, 0, 0) normal (1, 0, 0) x (0, 1, 0) in component "rightPalmRest1"
  line L0 (0, -15) -> (-79.0794, -15) construction
  line L1 (-10, -15) -> (-90, -15)
  line L2 (-90, -15) -> (-90, -3)
  line L3 (-90, -3) -> (-55.9723, 3)
  line L4 (-55.9723, 3) -> (-10.0816, 3)
  line L5 (-10.0816, 3) -> (-10, -15)
  point P0 (0, 3)
  point P1 (0, -15)
  dimension "d775" = 80
  dimension "d776" = 10
  dimension "d777" = 18
  dimension "d778" = 170
  dimension "d779" = 12
  constraint coincident P1 L0.start
  constraint horizontal L0
  constraint coincident L0 L1.start
  constraint parallel L0 L1
  constraint perpendicular L1 L2
  constraint perpendicular L2 L4
  measures "d775" distance of L1.start L1.end
  measures "d776" distance of P1 L1.start
  measures "d777" vertical distance of L1.start L4.end
  measures "d778" angle of L3 L4
  measures "d779" distance of L1.end L2.end
extrude "돌출1'''''''" add sketch "스케치1 (7)" against normal blind 99.45 separate body makes body 9 in component "rightPalmRest1"
sketch "스케치2 (6)" plane through (0, 0, -15) normal (0, 0, -1) x (1, 0, 0) in component "rightPalmRest1"
  line L0 (228.5, 10) -> (228.5, 90)
  line L1 (228.5, 90) -> (129.05, 90)
  line L2 (129.05, 90) -> (129.05, 10)
  line L3 (129.05, 10) -> (228.5, 10)
  line L4 (104.5156, 0) -> (228.5, 0)
  line L5 (228.5, 10) -> (228.5, 90)
  line L6 (129.05, 10) -> (129.05, 90)
  line L7 (228.5, 90) -> (228.5, 10)
  line L8 (129.05, 40) -> (124.05, 40)
  line L9 (124.05, 48) -> (129.05, 48)
  line L10 (129.05, 40) -> (129.05, 48)
  circle A0 centre (124.05, 44) radius 3.1
  circle A1 centre (124.05, 44) radius 1.5
  arc A2 (124.05, 48) -> (124.05, 40) centre (124.05, 44) ccw
  dimension "d788" = 30
  dimension "d870" = 6.2
  dimension "d871" = 3
  dimension "d872" = 4
  dimension "d873" = 8
  dimension "d874" = 5
  constraint coincident L0.end L1.start
  constraint coincident L0.start L3.end
  constraint horizontal L8
  constraint coincident L6 L9.end
  constraint perpendicular L6 L9
  constraint perpendicular L9 L10
  constraint concentric A0 A2
  constraint concentric A1 A2
  constraint equal L8 L9
  measures "d788" distance of L2.end L8.start
  measures "d870" diameter of A0
  measures "d871" diameter of A1
  measures "d872" radius of A2
  measures "d873" distance of L8.start L9.end
  measures "d874" distance of L8.start L8.end
extrude "돌출4''''" add sketch "스케치2 (6)" against normal blind 3 separate body contours L2 L6 L8 L9 L10 A2 | A0 makes body 10 in component "rightPalmRest1"
sketch "스케치1 (8)" plane through (129.05, 0, 0) normal (-1, 0, 0) x (0, -1, 0) in component "rightPalmRest2"
  line L0 (10.0816, 3) -> (10, -15)
  line L1 (55.9723, 3) -> (10.0816, 3)
  line L2 (90, -3) -> (55.9723, 3)
  line L3 (90, -15) -> (90, -3)
  line L4 (10, -15) -> (90, -15)
  line L5 (55.9723, 3) -> (10.0816, 3)
  line L6 (10.0816, 3) -> (10, -15)
  line L7 (10, -15) -> (90, -15)
  line L8 (90, -15) -> (90, -3)
  line L9 (90, -3) -> (55.9723, 3)
extrude "돌출1''''''''" add sketch "스케치1 (8)" along normal blind 99.05 separate body makes body 11 in component "rightPalmRest2"
sketch "스케치2 (7)" plane through (0, 0, -15) normal (0, 0, -1) x (1, 0, 0) in component "rightPalmRest2"
  line L0 (30, 55.9723) -> (30, 10.0816)
  line L1 (30, 90) -> (30, 55.9723)
  line L2 (129.05, 40) -> (124.05, 40)
  line L3 (124.05, 40) -> (129.05, 40)
  line L4 (124.05, 48) -> (129.05, 48)
  line L5 (129.05, 40) -> (129.05, 48)
  circle A0 centre (124.05, 44) radius 4
  circle A1 centre (124.05, 44) radius 3
  circle A2 centre (124.05, 44) radius 1.5
  dimension "d887" = 5
  dimension "d889" = 8
  dimension "d890" = 8
  dimension "d891" = 6
  dimension "d892" = 3
  constraint coincident L2.end L3.start
  constraint coincident L2.start L3.end
  constraint coincident L2.end A0
  constraint perpendicular L4 L5
  constraint vertical L2.end A0.centre
  constraint concentric A0 A1
  constraint concentric A0 A2
  measures "d887" distance of L4.start L4.end
  measures "d889" diameter of A0
  measures "d890" distance of L2.start L4.end
  measures "d891" diameter of A1
  measures "d892" diameter of A2
sketch "스케치1 (9)" plane through (-82.382, 0, 0) normal (1, 0, 0) x (0, 1, 0) in component "leftPalmRest2"
  line L0 (-90, -15) -> (-90, -3)
  line L1 (-90, -3) -> (-55.9723, 3)
  line L2 (-55.9723, 3) -> (-10.0816, 3)
  line L3 (-10.0816, 3) -> (-10, -15)
  line L4 (-10, -15) -> (-90, -15)
extrude "돌출1'''''''''" add sketch "스케치1 (9)" along normal blind 146.1125 separate body makes body 12 in component "leftPalmRest2"
draft "기울기1" angle -10 neutral plane through (-82.382, -10.0816, 3) pull (0, 0.99999, 0.004531) 1 faces at (63.7305, -51.9908, -9) on bodies 12 in component "leftPalmRest2"
draft "기울기1'" angle -10 neutral plane through (228.5, -10.0816, 3) pull (0, 0.99999, 0.004531) 1 faces at (228.5, -51.9908, -9) on bodies 9 in component "rightPalmRest1"
extrude "돌출6''" cut sketch "스케치2 (7)" against normal blind 3.1 contours L2 L3 L4 L5 A0 | A0 | A1 bodies 11 in component "rightPalmRest2"
extrude "돌출7''" cut 1 faces at (124.8658, -44.2169, -15) along direction (0, 0, 1) blind 12 on bodies 11 bodies 11 in component "rightPalmRest2"
move_face "면 간격띄우기2" offset -0.5 3 faces at (127.3833, -40, -12.9333) (120.404, -42.3549, -13.9667) (125.7167, -48, -12.9333) on bodies 11 in component "rightPalmRest2"
draft "기울기1''" angle -10 neutral plane through (129.05, -10.0816, 3) pull (0, 0.99999, 0.004531) 1 faces at (30, -51.9908, -9) on bodies 11 in component "rightPalmRest2"
fillet "모깎기2'" radius 5 5 edges at (34.0458, -33.0269, 3) (83.5708, -55.9723, 3) (41.0941, -72.9862, 0) (86.5732, -90, -3) (44.1012, -90, -9) on bodies 11 in component "rightPalmRest2"
fillet "모깎기2''" radius 5 5 edges at (171.7268, -90, -3) (174.7292, -55.9723, 3) (224.4542, -33.0269, 3) (217.4059, -72.9862, 0) (214.3988, -90, -9) on bodies 9 in component "rightPalmRest1"
move_face "면 간격띄우기1''" offset -0.1 1 faces at (122.6405, -43.487, -13) on bodies 10 in component "rightPalmRest1"
extrude "돌출6'''" cut sketch "스케치2 (6)" against normal blind 2 contours A0 bodies 10 in component "rightPalmRest1"
sketch "스케치1 (10)" plane through (0, 0, 0) normal (0, 0, 1) x (1, 0, 0)
sketch "스케치1 (11)" plane through (0, 0, 0) normal (0, 0, 1) x (1, 0, 0) in component "upper"
  line L0 (0, -100) -> (13, -100)
  line L1 (13, -100) -> (13, -113)
  line L2 (13, -113) -> (0, -113)
  line L3 (0, -113) -> (0, -100)
  dimension "d909" = 13
  dimension "d910" = 13
  dimension "d911" = 100
  constraint horizontal L0
  constraint vertical L1
  constraint horizontal L2
  constraint vertical L3
  constraint vertical L0.start origin
  measures "d909" distance of L0.start L0.end
  measures "d910" distance of L0.start L2.end
  measures "d911" distance of L0.start origin
extrude "돌출1''''''''''" add sketch "스케치1 (11)" along normal blind 7 draft 30 separate body makes body 13 in component "upper"
extrude "돌출2''''''" cut 1 faces at (4.3333, -108.6667, 0) along direction (0, 0, 1) blind 1 on bodies 13 bodies 13 in component "upper"
fillet "모깎기1'''''" radius 1 4 edges at (-2.0207, -115.0207, 3.5) (-2.0207, -97.9793, 3.5) (15.0207, -97.9793, 3.5) (15.0207, -115.0207, 3.5) on bodies 13 in component "upper"
move_body "이동1" bodies 12 to x (1, 0, 0) y (0, 1, 0) z (0, 0, 1) at (-65, 0, 0) in component "leftPalmRest2"
draft "기울기2" angle -10 neutral plane through (-147.382, -10.0816, 3) pull (0, 0.99999, 0.004531) 1 faces at (-147.382, -51.9908, -9) on bodies 12 in component "leftPalmRest2"
fillet "모깎기1''''''" radius 5 8 edges at (-74.3257, -90, -3) (-12.3636, -72.9862, 0) (-74.3257, -55.9723, 3) (-5.3153, -33.0269, 3) (-15.3707, -90, -9) (-143.3361, -33.0269, 3) (-136.2879, -72.9862, 0) (-133.2808, -90, -9) on bodies 12 in component "leftPalmRest2"
component "leftKey1" placed x (1, 0, 0) y (0, 1, 0) z (0, 0, 1) at (0, 0, 0)
component "leftBody1" placed x (1, 0, 0) y (0, 1, 0) z (0, 0, 1) at (0, 0, 0)
component "rightKey1" placed x (1, 0, 0) y (0, 1, 0) z (0, 0, 1) at (0, 0, 0)
component "rightKey2" placed x (1, 0, 0) y (0, 1, 0) z (0, 0, 1) at (0, 0, 0)
component "rightBody1" placed x (1, 0, 0) y (0, 1, 0) z (0, 0, 1) at (0, 0, 0)
component "rightBody2" placed x (1, 0, 0) y (0, 1, 0) z (0, 0, 1) at (0, 0, 0)
component "tempJoin" placed x (1, 0, 0) y (0, 1, 0) z (0, 0, 1) at (13.5824, 154.2275, -3.4182)
component "rightPalmRest1" placed x (1, 0, 0) y (0, 1, 0) z (0, 0, 1) at (0, 0, 0)
component "rightPalmRest2" placed x (1, 0, 0) y (0, 1, 0) z (0, 0, 1) at (0, 0, 0)
component "leftPalmRest2" placed x (1, 0, 0) y (0, 1, 0) z (0, 0, 1) at (0, 0, 0)
component "upper" placed x (1, 0, 0) y (0, 1, 0) z (0, 0, 1) at (0, 0, 0)
equation "keyHoleWidth = 14 mm"
equation "keyWidth = 19.05 mm"
equation "bodyMargin = 4 mm"
equation "boltKeyHole = 3.2 mm"
equation "boltBodyHole = 3 mm"
equation "d6 = boltKeyHole"
equation "bodyBoltCenterMargin = 3.1 mm"
equation "d8 = bodyBoltCenterMargin"
equation "d9 = bodyBoltCenterMargin"
equation "boltHead = 6 mm"
equation "d12 = boltKeyHole"
equation "d14 = bodyBoltCenterMargin"
equation "d15 = bodyBoltCenterMargin"
equation "d16 = ( 1.25 * 4 * keyWidth ) + ( 2.25 * keyWidth ) + bodyMargin * 2"
equation "d17 = ( 5 * keyWidth ) + bodyMargin * 2"
equation "d18 = keyHoleWidth"
equation "d19 = keyHoleWidth"
equation "keyMargin = ( keyWidth - keyHoleWidth ) / 2"
equation "d21 = ( keyWidth * 1.25 - keyHoleWidth ) / 2 + bodyMargin"
equation "d22 = bodyMargin + keyMargin"
equation "d25 = keyWidth * 1.25"
equation "d32 = keyHoleWidth"
equation "d33 = keyHoleWidth"
equation "d37 = keyWidth"
equation "d39 = keyHoleWidth"
equation "d40 = keyHoleWidth"
equation "d41 = ( keyWidth * 1.75 - keyHoleWidth ) / 2 + bodyMargin"
equation "d43 = keyHoleWidth"
equation "d44 = keyHoleWidth"
equation "d45 = ( keyWidth * 1.75 - keyHoleWidth ) / 2 + keyMargin"
equation "d48 = keyWidth"
equation "d50 = keyHoleWidth"
equation "d51 = keyHoleWidth"
equation "d52 = ( keyWidth * 1.5 - keyHoleWidth ) / 2 + bodyMargin"
equation "d53 = keyWidth"